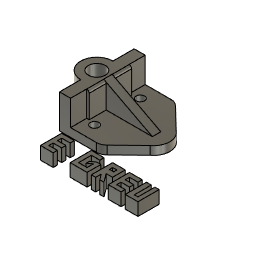
A3 (Autodesk Fusion 360 design; units mm, degrees)
Autodesk Fusion 360 part; units mm, degrees
sketch "Sketch1" plane through (0, 0, 0) normal (0, 0, 1) x (1, 0, 0)
  line L0 (15.1672, 44) -> (-33.5, 44)
  line L1 (-33.5, 44) -> (-33.5, -44)
  line L2 (-33.5, -44) -> (15.1672, -44)
  line L3 (24.1616, -31.7346) -> (25.7114, -33.7701) construction
  line L4 (44.6986, 15.349) -> (15.1672, 44)
  line L5 (44.6986, -15.349) -> (15.1672, -44)
  arc A0 (44.6986, -15.349) -> (44.6986, 15.349) centre (33.5, 0) ccw
  line L6 (-9.1664, -32) -> (-9.1664, -27) construction
  line L7 (-9.1664, 32) -> (-9.1664, 27) construction
  circle A1 centre (-9.1664, 27) radius 5
  circle A2 centre (-9.1664, -27) radius 5
  dimension "d2" = 88
  dimension "d3" = 38
  dimension "d7" = 10
  dimension "d8" = 10
  constraint horizontal L0
  constraint perpendicular L0 L1
  constraint parallel L0 L2
  constraint coincident L3 origin
  constraint perpendicular L2 L6
  constraint perpendicular L0 L7
  constraint coincident L7.end A1.centre
  constraint coincident L6.end A2.centre
  constraint coincident L5 L3.end
  constraint coincident A2 L6.start
  constraint coincident A1 L7.start
  measures "d2" distance of L0.end L1.end
  measures "d3" diameter of A0
  measures "d7" diameter of A1
  measures "d8" diameter of A2
sketch "Sketch2" plane through (0, 0, 0) normal (0, 0, 1) x (1, 0, 0)
  circle A0 centre (-33.5, 0) radius 9.5
  line L0 (-33.5, -19) -> (-33.5, -24)
  arc A1 (-33.5, 19) -> (-33.5, -19) centre (-33.5, 0) ccw
  line L1 (-33.5, -24) -> (-33.5, -19)
  line L2 (-33.5, 19) -> (-33.5, 24)
  line L3 (-33.5, -19) -> (-33.5, -9.5)
  line L4 (-33.5, 19) -> (-33.5, 9.5)
  dimension "d9" = 38
  dimension "d10" = 19
  constraint concentric A0 A1
  constraint collinear L1 L2
  constraint coincident A0 L3.end
  constraint parallel L0 L3
  constraint coincident A0 L4.end
  constraint parallel L2 L4
  measures "d9" diameter of A1
  measures "d10" diameter of A0
extrude "Extrude1" add sketch "Sketch2" sketch "Sketch1" along normal blind 10 contours A0 A1 L3 L4 of sketch 2 makes body 1
sketch "Sketch3" plane through (0, 0, 10) normal (0, 0, 1) x (-1, 0, 0)
  arc A0 (33.5, -19) -> (33.5, 19) centre (33.5, 0) ccw
  line L0 (33.5, 19) -> (33.5, 44)
  line L1 (33.5, 44) -> (-15.1672, 44)
  line L2 (-15.1672, 44) -> (-44.6986, 15.349)
  arc A1 (-44.6986, 15.349) -> (-44.6986, -15.349) centre (-33.5, 0) ccw
  line L3 (-44.6986, -15.349) -> (-15.1672, -44)
  line L4 (-15.1672, -44) -> (33.5, -44)
  line L5 (33.5, -44) -> (33.5, -19)
  circle A2 centre (9.1664, -27) radius 5
  circle A3 centre (9.1664, 27) radius 5
  line L6 (33.5, -9.5) -> (33.5, 9.5)
  arc A4 (33.5, -9.5) -> (33.5, 9.5) centre (33.5, 0) ccw
  line L7 (33.5, 44) -> (20.5, 44)
  line L8 (20.5, 44) -> (20.5, 5)
  line L9 (33.5, -44) -> (-33.5, -44) construction
  line L10 (-33.5, -44) -> (-33.5, 43.9899) construction
  line L11 (20.5, 5) -> (20.5, -44)
  line L12 (33.5, -44) -> (20.5, -44)
  line L13 (33.5, -44) -> (33.5, 44)
  dimension "d13" = 13
  dimension "d14" = 39
  dimension "d15" = 67
  constraint coincident L0.end L1.start
  constraint coincident L1 L7.end
  constraint perpendicular L7 L8
  constraint coincident L4.end L5.start
  constraint perpendicular L5 L9
  constraint perpendicular L9 L10
  constraint coincident L9 L11.end
  constraint perpendicular L9 L11
  measures "d13" distance of L0.end L7.end
  measures "d14" distance of L7.end L8.end
  measures "d15" distance of L4.end L9.end
extrude "Extrude2" add sketch "Sketch3" along normal blind 30 contours L0 L1 L4 L5 L6 L7 L8 L11 L12 L13 bodies 1
hole "Hole1" at (-33.5, 0, 40) direction (0, 0, -1) diameter 20 depth 45 tip angle 118 bodies 1
sketch "Sketch4" plane through (0, 0, 0) normal (0, 1, 0) x (1, 0, 0)
  line L0 (-20.5, -10) -> (37, -10)
  line L1 (37, -10) -> (-20.5, -40)
  line L2 (-20.5, -40) -> (-20.5, -10)
  constraint horizontal L0
  constraint perpendicular L0 L2
extrude "Extrude3" add sketch "Sketch4" along normal mid plane 10 bodies 1
extrude "Extrude4" add 1 faces at (-47.9833, -6.6983, 10) along direction (0, 0, 1) blind 30 on bodies 1 bodies 1
sketch "Sketch5" plane through (0, 0, 10) normal (0, 0, 1) x (-1, 0, 0)
  circle A0 centre (9.1664, 27) radius 5
  circle A1 centre (9.1664, -27) radius 5
  line L0 (20.5, -5) -> (-37, -5)
  line L1 (-37, -5) -> (-37, 5)
  line L2 (-37, 5) -> (20.5, 5)
  line L3 (20.5, 5) -> (20.5, 44)
  line L4 (20.5, 44) -> (-15.1672, 44)
  line L5 (-15.1672, 44) -> (-44.6986, 15.349)
  arc A2 (-44.6986, 15.349) -> (-44.6986, -15.349) centre (-33.5, 0) ccw
  line L6 (-44.6986, -15.349) -> (-15.1672, -44)
  line L7 (-15.1672, -44) -> (20.5, -44)
  line L8 (20.5, -44) -> (20.5, -5)
  line L9 (20.5, 5) -> (17.5, 5)
  line L10 (17.5, 5) -> (17.5, 25)
  line L11 (17.5, 25) -> (20.5, 25)
  line L12 (20.5, 25) -> (20.5, 5)
  line L13 (20.5, -5) -> (17.5, -5)
  line L14 (17.5, -5) -> (17.5, -25)
  line L15 (17.5, -25) -> (20.5, -25)
  line L16 (20.5, -25) -> (20.5, -5)
  dimension "d26" = 3
  dimension "d27" = 20
  dimension "d28" = 3
  dimension "d29" = 20
  constraint coincident L2.end L3.start
  constraint perpendicular L3 L9
  constraint perpendicular L9 L10
  constraint coincident L3 L11.end
  constraint perpendicular L3 L11
  constraint coincident L0.start L8.end
  constraint coincident L0 L13.end
  constraint perpendicular L13 L14
  constraint coincident L8 L15.end
  constraint perpendicular L8 L15
  measures "d26" distance of L2.end L9.end
  measures "d27" distance of L9.end L10.end
  measures "d28" distance of L0.start L13.end
  measures "d29" distance of L13.end L14.end
extrude "Extrude5" add sketch "Sketch5" along normal blind 30 contours L0 L8 L13 L14 L15 L16 | L2 L3 L9 L10 L11 L12 bodies 1
fillet "Fillet1" radius 2.9 1 edges at (-17.5, -15, 40) on bodies 1
fillet "Fillet2" radius 2.9 1 edges at (-17.5, 15, 40) on bodies 1
sketch "Sketch6" plane through (0, 0, 0) normal (0, 0, 1) x (1, 0, 0)
  line L0 (-15, -60) -> (0, -60)
  line L1 (0, -60) -> (0, -65)
  line L2 (0, -65) -> (-10, -65)
  line L3 (-10, -65) -> (-10, -70)
  line L4 (-10, -70) -> (0, -70)
  line L5 (0, -70) -> (0, -75)
  line L6 (0, -75) -> (-10, -75)
  line L7 (-10, -75) -> (-10, -80)
  line L8 (-10, -80) -> (0, -80)
  line L9 (0, -80) -> (0, -85)
  line L10 (0, -85) -> (-15, -85)
  line L11 (-15, -85) -> (-15, -60)
  line L12 (20, -60) -> (35, -60)
  line L13 (35, -60) -> (35, -65)
  line L14 (35, -65) -> (27.5, -65)
  line L15 (27.5, -65) -> (25, -65)
  line L16 (25, -65) -> (25, -80)
  line L17 (25, -80) -> (35, -80)
  line L18 (35, -80) -> (35, -72.5)
  line L19 (35, -72.5) -> (30, -76.25)
  line L20 (30, -76.25) -> (30, -72.5)
  line L21 (30, -72.5) -> (35, -68.75)
  line L22 (35, -68.75) -> (40, -68.75)
  line L23 (40, -68.75) -> (40, -85)
  line L24 (40, -85) -> (20, -85)
  line L25 (20, -85) -> (20, -60)
  line L26 (45, -85) -> (45, -60)
  line L27 (45, -60) -> (60, -60)
  line L28 (60, -60) -> (60, -75)
  line L29 (60, -75) -> (52.5, -75)
  line L30 (52.5, -75) -> (60, -85)
  line L31 (60, -85) -> (55, -85)
  line L32 (55, -85) -> (50.093, -78.4573)
  line L33 (50.093, -78.4573) -> (50.093, -85)
  line L34 (50.093, -85) -> (45, -85)
  line L35 (50.093, -65) -> (50.093, -68.75)
  line L36 (50.093, -68.75) -> (55, -68.75)
  line L37 (55, -68.75) -> (55, -65)
  line L38 (55, -65) -> (50.093, -65)
  line L39 (65, -85) -> (65, -60)
  line L40 (65, -60) -> (80, -60)
  line L41 (80, -60) -> (80, -65)
  line L42 (80, -65) -> (70, -65)
  line L43 (70, -65) -> (70, -70)
  line L44 (70, -70) -> (80, -70)
  line L45 (80, -70) -> (80, -75)
  line L46 (80, -75) -> (70, -75)
  line L47 (70, -75) -> (70, -80)
  line L48 (70, -80) -> (80, -80)
  line L49 (80, -80) -> (80, -85)
  line L50 (80, -85) -> (65, -85)
  line L51 (85, -60) -> (85, -85)
  line L52 (85, -85) -> (100, -85)
  line L53 (100, -85) -> (100, -60)
  line L54 (100, -60) -> (95, -60)
  line L55 (95, -60) -> (95, -80)
  line L56 (85, -60) -> (90.7249, -60)
  line L57 (90.7249, -60) -> (90.7249, -80)
  line L58 (90.7249, -80) -> (95, -80)
  constraint horizontal L0
  constraint perpendicular L0 L1
  constraint perpendicular L1 L2
  constraint perpendicular L2 L3
  constraint perpendicular L3 L4
  constraint perpendicular L4 L5
  constraint perpendicular L5 L6
  constraint perpendicular L6 L7
  constraint perpendicular L5 L8
  constraint perpendicular L8 L9
  constraint perpendicular L9 L10
  constraint perpendicular L0 L11
  constraint perpendicular L1 L12
  constraint perpendicular L12 L13
  constraint perpendicular L13 L14
  constraint perpendicular L13 L15
  constraint perpendicular L14 L16
  constraint perpendicular L16 L17
  constraint perpendicular L17 L18
  constraint perpendicular L17 L20
  constraint parallel L19 L21
  constraint perpendicular L18 L22
  constraint perpendicular L22 L23
  constraint perpendicular L16 L24
  constraint perpendicular L12 L25
  constraint perpendicular L22 L26
  constraint perpendicular L26 L27
  constraint perpendicular L27 L28
  constraint perpendicular L26 L29
  constraint parallel L29 L31
  constraint parallel L30 L32
  constraint perpendicular L29 L33
  constraint perpendicular L26 L34
  constraint perpendicular L22 L35
  constraint perpendicular L26 L36
  constraint perpendicular L36 L37
  constraint perpendicular L35 L38
  constraint perpendicular L27 L39
  constraint perpendicular L39 L40
  constraint perpendicular L40 L41
  constraint perpendicular L41 L42
  constraint perpendicular L42 L43
  constraint perpendicular L43 L44
  constraint perpendicular L42 L45
  constraint perpendicular L45 L46
  constraint perpendicular L46 L47
  constraint perpendicular L47 L48
  constraint perpendicular L48 L49
  constraint perpendicular L39 L50
  constraint perpendicular L46 L51
  constraint perpendicular L45 L52
  constraint perpendicular L52 L53
  constraint perpendicular L45 L54
  constraint perpendicular L54 L55
  constraint perpendicular L51 L56
  constraint perpendicular L56 L57
  constraint perpendicular L55 L58
extrude "Extrude6" add sketch "Sketch6" along normal blind 15 separate body makes body 2 at (45, -76.6667, 5) makes body 3 at (20, -76.6667, 5) makes body 4 at (65, -76.6667, 5) makes body 5 at (-15, -76.6667, 5) makes body 6 at (100, -76.6667, 5)
fillet "Fillet3" radius 13 1 edges at (15.1672, -44, 5) on bodies 1
fillet "Fillet4" radius 13 1 edges at (15.1672, 44, 5) on bodies 1
equation "d21 = 4.992E-07 mm"
